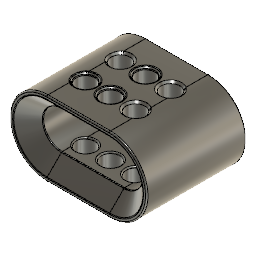
v3 (Autodesk Fusion 360 design; units mm, degrees)
Autodesk Fusion 360 part; units mm, degrees
sketch "Sketch4" plane through (0, 0, 0) normal (0, 1, 0) x (1, 0, 0) in component "Standur_vol2"
  line L0 (-25, -30) -> (25, -30)
  line L1 (25, 30) -> (-25, 30)
  line L2 (1.75, 0) -> (22.5, 0)
  line L3 (0, -1.75) -> (0, -22.5)
  arc A0 (-25, 30) -> (-25, -30) centre (-25, 0) ccw
  arc A1 (25, -30) -> (25, 30) centre (25, 0) ccw
  line L4 (-25, -15) -> (25, -15)
  arc A2 (25, -15) -> (25, 15) centre (25, 0) ccw
  line L5 (25, 15) -> (-25, 15)
  arc A3 (-25, 15) -> (-25, -15) centre (-25, 0) ccw
  point P0 (75.7145, 35)
  point P1 (75.7145, -35)
  dimension "d107" = 60
  dimension "d108" = 50
  dimension "d109" = -15
  constraint horizontal L0
  constraint horizontal L1
  constraint tangent L0 A0
  constraint tangent L1 A0
  constraint symmetric L0 L1 L2
  constraint symmetric L3 A0 A1
  measures "d107" distance of L0 L1
  measures "d108" distance of A0.centre A1.centre
extrude "Extrude4" add sketch "Sketch4" along normal mid plane 80 in component "Standur_vol2"
sketch "Sketch5" plane through (0, 0, 30) normal (0, 0, 1) x (-1, 0, 0) in component "Standur_vol2"
  line L0 (-25, 40) -> (-25, -40)
  line L1 (-25, -40) -> (25, -40)
  line L2 (25, -40) -> (25, 40)
  line L3 (25, 40) -> (-25, 40)
  circle A0 centre (0, 14) radius 7.5
  line L4 (0, -28.1943) -> (0, 29) construction
  line L5 (0, -1.75) -> (0, -22.5)
  dimension "d112" = 15
  dimension "d113" = 14
  constraint vertical L4
  constraint coincident A0.centre L4
  constraint collinear L4 L5
  measures "d112" diameter of A0
  measures "d113" distance of origin A0.centre
extrude "Extrude5" cut sketch "Sketch5" against normal up to surface (65 mm away) contours A0 in component "Standur_vol2"
pattern_linear "R-Pattern2" count 3 spacing 20 along (-1, 0, 0) both ways count 2 spacing 28 along (0, 1, 0) of "Extrude5" in component "Standur_vol2"
chamfer "Chamfer3" distance 12 angle 45 8 edges at (-40, -40, 0) (0, -40, 15) (40, -40, 0) (0, -40, -15) (-40, 40, 0) (0, 40, -15) (40, 40, 0) (0, 40, 15) measured on face at (8.3333, -40, -20) measured on face at (8.3333, -40, -20) measured on face at (8.3333, -40, -20) measured on face at (8.3333, -40, -20) measured on face at (8.3333, 40, -20) measured on face at (8.3333, 40, -20) measured on face at (8.3333, 40, -20) measured on face at (8.3333, 40, -20) in component "Standur_vol2"
chamfer "Chamfer4" distance 1.5 angle 45 2 edges at (6.9925, 11.2879, 30) (6.9925, -16.7121, 30) measured on face at (0.1868, 33.8263, 30) measured on face at (0.1868, 33.8263, 30) in component "Standur_vol2"
fillet "Fillet7" radius 1 18 edges at (55, 40, 0) (0, 40, -30) (-55, 40, 0) (0, 40, 30) (52, 40, 0) (0, 40, -27) (-52, 40, 0) (0, 40, 27) (55, -40, 0) (0, -40, 30) (-55, -40, 0) (0, -40, -30) (52, -40, 0) (0, -40, 27) (-52, -40, 0) (0, -40, -27) (6.9925, 11.2879, -15) (6.9925, -16.7121, -15) in component "Standur_vol2"
fillet "Fillet8" radius 1 14 edges at (-40, -28, 0) (0, -28, 15) (40, -28, 0) (0, -28, -15) (0, -28, -15) (0, -28, -15) (0, -28, -15) (0, 28, 15) (-40, 28, 0) (0, 28, -15) (0, 28, -15) (0, 28, -15) (0, 28, -15) (40, 28, 0) in component "Standur_vol2"
sketch "Sketch8" plane through (0, 0, -15) normal (0, 0, 1) x (-1, 0, 0)
  line L0 (-25, -27.5858) -> (25, -27.5858)
  line L1 (25, 27.5858) -> (-25, 27.5858)
  line L2 (-25, 27.5858) -> (-25, 19.5902)
  circle A0 centre (0, -14) radius 8.5
  circle A1 centre (0, 14) radius 8.5
  circle A2 centre (20, -14) radius 5
  arc A3 (-25, 8.4098) -> (-25, 19.5902) centre (-20, 14) ccw
  line L3 (25, -27.5858) -> (25, -19.5902)
  line L4 (25, 19.5902) -> (25, 27.5858)
  arc A4 (25, -8.4098) -> (25, -19.5902) centre (20, -14) ccw
  line L5 (-25, 8.4098) -> (-25, -8.4098)
  line L6 (-25, -19.5902) -> (-25, -27.5858)
  line L7 (25, -8.4098) -> (25, 8.4098)
  arc A5 (25, 19.5902) -> (25, 8.4098) centre (20, 14) ccw
  arc A6 (-25, -19.5902) -> (-25, -8.4098) centre (-20, -14) ccw
  dimension "d174" = 10
  measures "d174" diameter of A2
chamfer "Chamfer6" distance 1.5 angle 45 4 edges at (-12.5, -14, 30) (-12.5, 14, 30) (12.5, 14, 30) (12.5, -14, 30) in component "Standur_vol2"
fillet "Fillet13" radius 1 6 edges at (-11, -14, 30) (8.3909, 17.2545, 30) (6.9925, 11.2879, 28.5) (-12.5, -14, 28.5) (8.3909, -10.7455, 30) (6.9925, -16.7121, 28.5) in component "Standur_vol2"
fillet "Fillet14" radius 1 8 edges at (-12.5, -14, -15) (-27.5, -14, -14.7902) (12.5, -14, -15) (27.5, -14, -14.7902) (-12.5, 14, -15) (-27.5, 14, -14.7902) (12.5, 14, -15) (27.5, 14, -14.7902) in component "Standur_vol2"
component "Standur_vol2" placed x (1, 0, 0) y (0, 1, 0) z (0, 0, 1) at (0, 0, 0)
equation "Lengd = 70 mm + 2 * Milli_hringja"
equation "Hæð = 60 mm"
equation "Dýpt = 80 mm"
equation "Veggjaþykkt = 15 mm"
equation "Milli_hringja = 20 mm"
equation "Gat_bursta = 15 mm"
equation "Curve = 15 mm"
equation "komast_út = 10 mm"
equation "Lengd_fra_brun = 40 mm"
equation "gat_oní = 20 mm"
equation "chamfer = 10 mm"
equation "d107 = Hæð"
equation "d108 = Lengd - Hæð"
equation "d109 = -Veggjaþykkt"
equation "d110 = Dýpt / 2"
equation "d112 = Gat_bursta"
equation "d113 = Bil_þvert"
equation "d114 = -gat_oní"
equation "d118 = Milli_hringja"
equation "d119 = Bil_þvert * 2"
equation "d120 = Veggjaþykkt - Brún"
equation "Brún = 3 mm"
equation "Bil_þvert = 14 mm"
equation "gat = 10 mm"
equation "Vessel_f_vatn = 10 mm"
